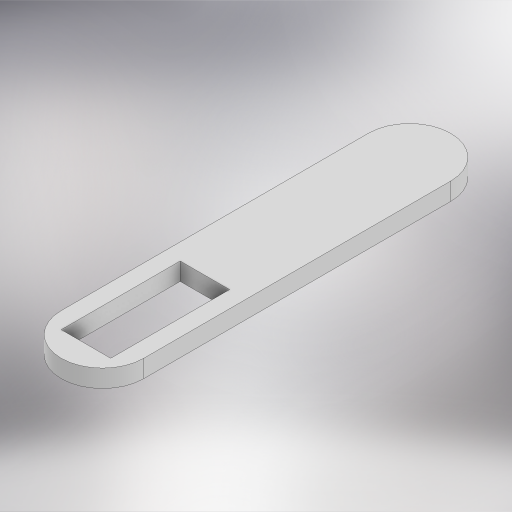
# Autodesk Inventor part: arm
Saved by Autodesk Inventor 2024 (Build 280153000, 153)
## iProperties
Created: 2023-10-08
Part Number: arm
Material: Generic
Document SubType Name: Modeling
Designer: byrne
Density: 1 g/cm^3
Appearance: Default
Author: byrne
Autodesk Inventor part; units mm, degrees
ref_plane "YZ Plane" through (0, 0, 0) normal (1, 0, 0) x (0, 1, 0)
ref_plane "XZ Plane" through (0, 0, 0) normal (0, 1, 0) x (-1, 0, 0)
ref_plane "XY Plane" through (0, 0, 0) normal (0, 0, 1) x (1, 0, 0)
sketch "Sketch1" plane through (0, 0, 0) normal (0, 1, 0) x (-1, 0, 0)
  arc A0 (1.4918, 12.1563) -> (-1.4918, 12.1563) centre (0, 12) ccw
  arc A1 (-1.4918, -12.1563) -> (1.4918, -12.1563) centre (0, -12) ccw
  line L0 (0, -12) -> (0, 12) construction
  line L1 (-2.735, 0.2865) -> (-1.4918, 12.1563)
  line L2 (1.4918, -12.1563) -> (2.735, -0.2865)
  line L3 (-1.4918, -12.1563) -> (-2.735, -0.2865)
  line L4 (2.735, 0.2865) -> (1.4918, 12.1563)
  arc A2 (-2.735, 0.2865) -> (-2.735, -0.2865) centre (0, 0) ccw
  arc A3 (2.735, -0.2865) -> (2.735, 0.2865) centre (0, 0) ccw
  line L5 (2.75, 0) -> (-2.75, 0) construction
  line L6 (-3.0334, -0.3177) -> (-1.7902, -12.1875)
  arc A4 (-1.7902, -12.1875) -> (1.7902, -12.1875) centre (0, -12) ccw
  line L7 (1.7902, -12.1875) -> (3.0334, -0.3177)
  arc A5 (3.0334, -0.3177) -> (3.0334, 0.3177) centre (0, 0) ccw
  line L8 (3.0334, 0.3177) -> (1.7902, 12.1875)
  arc A6 (1.7902, 12.1875) -> (-1.7902, 12.1875) centre (0, 12) ccw
  line L9 (-1.7902, 12.1875) -> (-3.0334, 0.3177)
  arc A7 (-3.0334, 0.3177) -> (-3.0334, -0.3177) centre (0, 0) ccw
  line L10 (-4.25, 27.45) -> (4.25, 27.45)
  line L11 (4.25, 27.45) -> (4.25, 48.45)
  line L12 (4.25, 48.45) -> (-4.25, 48.45)
  line L13 (-4.25, 48.45) -> (-4.25, 27.45)
  line L14 (0, -16.975) -> (0, 53.0999) construction
  line L15 (-7.425, -9.55) -> (-7.425, 45.6749)
  line L16 (7.425, 45.6749) -> (7.425, -9.55)
  arc A8 (-7.425, -9.55) -> (7.425, -9.55) centre (0, -9.55) ccw
  arc A9 (7.425, 45.6749) -> (-7.425, 45.6749) centre (0, 45.6749) ccw
  line L17 (4.45, 48.65) -> (4.45, 27.25)
  line L18 (4.45, 27.25) -> (-4.45, 27.25)
  line L19 (-4.45, 27.25) -> (-4.45, 48.65)
  line L20 (-4.45, 48.65) -> (4.45, 48.65)
  point P0 (0, 0)
  point P1 (0, 27.45)
  point P2 (0, 44.45)
  point P3 (0, 18.0624)
  point P4 (0, -13.8)
  point P5 (0, -16.975)
  dimension "d5" = 3
  dimension "d6" = 3
  dimension "d7" = 24
  dimension "d8" = 5.5
  dimension "d9" = 0.3
  dimension "d10" = 8.5
  dimension "d11" = 21
  dimension "d12" = 4
  dimension "d13" = 44.45
  dimension "d14" = 3.175
  dimension "d15" = 3.175
  dimension "d16" = 0.2
  constraints: 44 end point, 26 point on circle, 12 tangent, 10 centre point, 5 midpoint, 5 parallel, 2 perpendicular, 2 point on line, 2 vertical, 1 coincident, 1 collinear, 1 horizontal, 1 vertical alignment, 11 other
  measures "d5" diameter of A0
  measures "d6" diameter of A1
  measures "d7" distance of L0.start L0.end
  measures "d8" distance of L5.start L5.end
  measures "d9" distance between parallel lines of L3 L6
  measures "d10" distance of L12.end L11.end
  measures "d11" distance of L11.end L10.end
  measures "d12" distance from line of L12 point (0, 44.45)
  measures "d13" distance of point (0, 44.45) A2.centre
  measures "d14" distance between parallel lines of L15 L13
  measures "d15" distance of point (0, -13.8) point (0, -16.975)
  measures "d16" distance between parallel lines of L11 L17
extrude "Extrusion1" add sketch "Sketch1" along normal blind 1.5875 contours L15 A9 L16 A8
sketch "Sketch2" plane through (0, 1.5875, 0) normal (0, 1, 0) x (1, 0, 0)
  line L0 (7.425, -45.6749) -> (7.425, 9.55) projected
  arc A0 (7.425, 9.55) -> (-7.425, 9.55) centre (0, 9.55) ccw projected
  line L1 (-7.425, 9.55) -> (-7.425, -45.6749) projected
  arc A1 (-7.425, -45.6749) -> (7.425, -45.6749) centre (0, -45.6749) ccw projected
  line L2 (-4.45, -48.65) -> (-4.45, -27.25) projected
  line L3 (-4.45, -27.25) -> (4.45, -27.25) projected
  line L4 (4.45, -27.25) -> (4.45, -48.65) projected
  line L5 (4.45, -48.65) -> (-4.45, -48.65) projected
  arc A2 (3.0334, -0.3177) -> (3.0334, 0.3177) centre (0, 0) ccw projected
  line L6 (3.0334, -0.3177) -> (1.7902, -12.1875) projected
  arc A3 (-1.7902, -12.1875) -> (1.7902, -12.1875) centre (0, -12) ccw projected
  line L7 (-1.7902, -12.1875) -> (-3.0334, -0.3177) projected
  arc A4 (-3.0334, 0.3177) -> (-3.0334, -0.3177) centre (0, 0) ccw projected
  line L8 (-3.0334, 0.3177) -> (-1.7902, 12.1875) projected
  arc A5 (1.7902, 12.1875) -> (-1.7902, 12.1875) centre (0, 12) ccw projected
  line L9 (1.7902, 12.1875) -> (3.0334, 0.3177) projected
extrude "Extrusion2" add sketch "Sketch2" along normal blind 1.5875 contours A1 L1 A0 L0 | L6 A3 L7 A4 L8 A5 L9 A2
body "Solid1"
